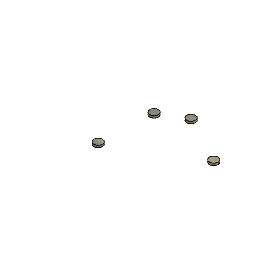
Mounting Base Magnets (Autodesk Fusion 360 design; units mm, degrees)
Autodesk Fusion 360 part; units mm, degrees
sketch "Sketch1" plane through (-0.1196, 0, 7.5625) normal (0, -1, 0) x (0.866025, 0, 0.5) in component "Magnet 1"
  circle A0 centre (26.3643, 45.4252) radius 3.7465
  arc A1 (44.7183, 43.9659) -> (15.1751, 60.8044) centre (-3.6777, -6.6091) ccw
  line L0 (15.1751, 60.8044) -> (16.1175, 64.6499)
  line L1 (16.1175, 64.6499) -> (8.0998, 66.6149)
  line L2 (8.0998, 66.6149) -> (7.1419, 62.7066)
  arc A2 (5.8468, 64.9166) -> (7.1419, 62.7066) centre (8.3868, 64.9206) ccw
  line L3 (5.8468, 64.9166) -> (5.7518, 125.1691)
  spline S0 degree 3 poles (7.7764, 127.6603) (7.4526, 127.5932) (7.1449, 127.4634) (6.5966, 127.0934) (6.3612, 126.8565) (6.0393, 126.3733) (5.9322, 126.146) (5.7879, 125.6676) (5.7514, 125.419) (5.7518, 125.1691) knots 0 0 0 0 0.099224 0.099224 0.198447 0.198447 0.273413 0.273413 0.348379 0.348379 0.348379 0.348379
  spline S1 degree 3 poles (7.7764, 127.6603) (8.1399, 127.7356) (8.4987, 127.8355) (9.8415, 128.3097) (10.758, 128.8464) (12.3456, 130.2408) (13.0009, 131.0881) (13.8928, 132.8639) (14.1662, 133.7539) (14.2925, 134.7176) (14.2982, 134.7643) (14.3035, 134.8111) knots 0.204697 0.204697 0.204697 0.204697 0.31653 0.31653 0.631913 0.631913 0.94989 0.94989 1.226398 1.226398 1.24048 1.24048 1.24048 1.24048
  spline S2 degree 3 poles (17.1425, 137.0446) (16.8143, 137.0856) (16.4812, 137.0622) (15.8428, 136.889) (15.5436, 136.7408) (15.0188, 136.3382) (14.7982, 136.0875) (14.5437, 135.6501) (14.4714, 135.4899) (14.3611, 135.157) (14.3233, 134.9853) (14.3035, 134.8111) knots 0 0 0 0 0.099224 0.099224 0.198447 0.198447 0.297671 0.297671 0.350269 0.350269 0.402867 0.402867 0.402867 0.402867
  spline S3 degree 3 poles (17.1425, 137.0446) (33.9368, 134.9438) (50.2112, 129.7725) (74.382, 116.8419) (83.022, 110.8694) (98.0523, 97.7289) (104.5331, 90.7629) (110.2478, 83.1896) knots 0.297104 0.297104 0.297104 0.297104 5.379677 5.379677 8.520913 8.520913 11.369176 11.369176 11.369176 11.369176
  spline S4 degree 3 poles (109.748, 79.6305) (110.0123, 79.8295) (110.2351, 80.0781) (110.5729, 80.6468) (110.6847, 80.9615) (110.7813, 81.6159) (110.7652, 81.9494) (110.6446, 82.4364) (110.5868, 82.5978) (110.4397, 82.9065) (110.3508, 83.0531) (110.2478, 83.1896) knots 0 0 0 0 0.099224 0.099224 0.198447 0.198447 0.297671 0.297671 0.34897 0.34897 0.400269 0.400269 0.400269 0.400269
  spline S5 degree 3 poles (109.748, 79.6305) (109.5783, 79.5028) (109.4134, 79.3683) (108.4318, 78.5028) (107.763, 77.6215) (106.8164, 75.6696) (106.5411, 74.6194) (106.4224, 72.7055) (106.4994, 71.8624) (106.7528, 70.8428) (106.8106, 70.6426) (106.8759, 70.4451) knots 0.2561 0.2561 0.2561 0.2561 0.320016 0.320016 0.648768 0.648768 0.972242 0.972242 1.225878 1.225878 1.288694 1.288694 1.288694 1.288694
  spline S6 degree 3 poles (105.7308, 67.4462) (106.0175, 67.6111) (106.2693, 67.8304) (106.6745, 68.3533) (106.8241, 68.6518) (106.979, 69.2114) (107.0097, 69.4607) (106.9974, 69.9603) (106.9544, 70.2079) (106.8759, 70.4451) knots 0 0 0 0 0.099224 0.099224 0.198447 0.198447 0.273411 0.273411 0.348375 0.348375 0.348375 0.348375
  line L4 (105.7308, 67.4462) -> (53.5032, 37.4022)
  arc A3 (50.3987, 37.8508) -> (53.5032, 37.4022) centre (52.2366, 39.6039) ccw
  line L5 (50.3987, 37.8508) -> (53.2273, 41.3906)
  line L6 (53.2273, 41.3906) -> (46.7784, 46.5439)
  line L7 (46.7784, 46.5439) -> (44.7183, 43.9659)
  circle A4 centre (114.2687, 72.6834) radius 4
  circle A5 centre (44.0521, 36.0691) radius 4
  circle A6 centre (6.0236, 135.1787) radius 4
  circle A7 centre (9.4154, 56.0666) radius 4
  arc A8 (129.4312, 70.2414) -> (-3.6777, 147.0918) centre (-3.6777, -6.6091) ccw
  line L8 (-3.6777, 147.0918) -> (-3.6777, 51.126)
  line L9 (-3.6777, 51.126) -> (46.3223, 22.2584)
  line L10 (46.3223, 22.2584) -> (129.4312, 70.2414)
  circle A9 centre (44.0521, 36.0691) radius 6.3691
  dimension "d669" = 12.7381
  constraint concentric A5 A9
  measures "d669" diameter of A9
extrude "Extrude1" add sketch "Sketch1" along normal blind 3.175 contours A5 | A9 makes body 1 in component "Magnet 1"
sketch "Sketch2" plane through (0, 0, 0) normal (0, 1, 0) x (-1, 0, 0) in component "Magnet 1"
  circle A0 centre (-19.9962, 60.8253) radius 6.3691
  circle A1 centre (-19.9962, 60.8253) radius 1.8288
  dimension "d672" = 3.6576
  constraint concentric A0 A1
  measures "d672" diameter of A1
sketch "Sketch3" plane through (0, 0, 0) normal (0, 1, 0) x (-1, 0, 0) in component "Magnet 1"
  circle A0 centre (-19.9962, 60.8253) radius 6.3691
  circle A1 centre (-44.0521, 36.0691) radius 3.683
  dimension "d675" = 7.366
  measures "d675" diameter of A1
sketch "Sketch1 (2)" plane through (-0.1196, -0.0025, 7.5625) normal (0, -1, 0) x (0.866025, 0, 0.5) in component "Magnet 1 (1)"
  circle A0 centre (26.3643, 45.4252) radius 3.7465
  arc A1 (44.7183, 43.9659) -> (15.1751, 60.8044) centre (-3.6777, -6.6091) ccw
  line L0 (15.1751, 60.8044) -> (16.1175, 64.6499)
  line L1 (16.1175, 64.6499) -> (8.0998, 66.6149)
  line L2 (8.0998, 66.6149) -> (7.1419, 62.7066)
  arc A2 (5.8468, 64.9166) -> (7.1419, 62.7066) centre (8.3868, 64.9206) ccw
  line L3 (5.8468, 64.9166) -> (5.7518, 125.1691)
  spline S0 degree 3 poles (7.7764, 127.6603) (7.4526, 127.5932) (7.1449, 127.4634) (6.5966, 127.0934) (6.3612, 126.8565) (6.0393, 126.3733) (5.9322, 126.146) (5.7879, 125.6676) (5.7514, 125.419) (5.7518, 125.1691) knots 0 0 0 0 0.099224 0.099224 0.198447 0.198447 0.273413 0.273413 0.348379 0.348379 0.348379 0.348379
  spline S1 degree 3 poles (7.7764, 127.6603) (8.1399, 127.7356) (8.4987, 127.8355) (9.8415, 128.3097) (10.758, 128.8464) (12.3456, 130.2408) (13.0009, 131.0881) (13.8928, 132.8639) (14.1662, 133.7539) (14.2925, 134.7176) (14.2982, 134.7643) (14.3035, 134.8111) knots 0.204697 0.204697 0.204697 0.204697 0.31653 0.31653 0.631913 0.631913 0.94989 0.94989 1.226398 1.226398 1.24048 1.24048 1.24048 1.24048
  spline S2 degree 3 poles (17.1425, 137.0446) (16.8143, 137.0856) (16.4812, 137.0622) (15.8428, 136.889) (15.5436, 136.7408) (15.0188, 136.3382) (14.7982, 136.0875) (14.5437, 135.6501) (14.4714, 135.4899) (14.3611, 135.157) (14.3233, 134.9853) (14.3035, 134.8111) knots 0 0 0 0 0.099224 0.099224 0.198447 0.198447 0.297671 0.297671 0.350269 0.350269 0.402867 0.402867 0.402867 0.402867
  spline S3 degree 3 poles (17.1425, 137.0446) (33.9368, 134.9438) (50.2112, 129.7725) (74.382, 116.8419) (83.022, 110.8694) (98.0523, 97.7289) (104.5331, 90.7629) (110.2478, 83.1896) knots 0.297104 0.297104 0.297104 0.297104 5.379677 5.379677 8.520913 8.520913 11.369176 11.369176 11.369176 11.369176
  spline S4 degree 3 poles (109.748, 79.6305) (110.0123, 79.8295) (110.2351, 80.0781) (110.5729, 80.6468) (110.6847, 80.9615) (110.7813, 81.6159) (110.7652, 81.9494) (110.6446, 82.4364) (110.5868, 82.5978) (110.4397, 82.9065) (110.3508, 83.0531) (110.2478, 83.1896) knots 0 0 0 0 0.099224 0.099224 0.198447 0.198447 0.297671 0.297671 0.34897 0.34897 0.400269 0.400269 0.400269 0.400269
  spline S5 degree 3 poles (109.748, 79.6305) (109.5783, 79.5028) (109.4134, 79.3683) (108.4318, 78.5028) (107.763, 77.6215) (106.8164, 75.6696) (106.5411, 74.6194) (106.4224, 72.7055) (106.4994, 71.8624) (106.7528, 70.8428) (106.8106, 70.6426) (106.8759, 70.4451) knots 0.2561 0.2561 0.2561 0.2561 0.320016 0.320016 0.648768 0.648768 0.972242 0.972242 1.225878 1.225878 1.288694 1.288694 1.288694 1.288694
  spline S6 degree 3 poles (105.7308, 67.4462) (106.0175, 67.6111) (106.2693, 67.8304) (106.6745, 68.3533) (106.8241, 68.6518) (106.979, 69.2114) (107.0097, 69.4607) (106.9974, 69.9603) (106.9544, 70.2079) (106.8759, 70.4451) knots 0 0 0 0 0.099224 0.099224 0.198447 0.198447 0.273411 0.273411 0.348375 0.348375 0.348375 0.348375
  line L4 (105.7308, 67.4462) -> (53.5032, 37.4022)
  arc A3 (50.3987, 37.8508) -> (53.5032, 37.4022) centre (52.2366, 39.6039) ccw
  line L5 (50.3987, 37.8508) -> (53.2273, 41.3906)
  line L6 (53.2273, 41.3906) -> (46.7784, 46.5439)
  line L7 (46.7784, 46.5439) -> (44.7183, 43.9659)
  circle A4 centre (114.2687, 72.6834) radius 4
  circle A5 centre (44.0521, 36.0691) radius 4
  circle A6 centre (6.0236, 135.1787) radius 4
  circle A7 centre (9.4154, 56.0666) radius 4
  arc A8 (129.4312, 70.2414) -> (-3.6777, 147.0918) centre (-3.6777, -6.6091) ccw
  line L8 (-3.6777, 147.0918) -> (-3.6777, 51.126)
  line L9 (-3.6777, 51.126) -> (46.3223, 22.2584)
  line L10 (46.3223, 22.2584) -> (129.4312, 70.2414)
  circle A9 centre (44.0521, 36.0691) radius 6.3691
  dimension "d669_1" = 12.7381
  constraint concentric A5 A9
  measures "d669_1" diameter of A9
extrude "Extrude1'" add sketch "Sketch1 (2)" along normal blind 3.175 separate body contours A5 | A9 makes body 2 in component "Magnet 1 (1)"
sketch "Sketch2 (2)" plane through (0, -0.0025, 0) normal (0, 1, 0) x (-1, 0, 0) in component "Magnet 1 (1)"
  circle A0 centre (-19.9962, 60.8253) radius 6.3691
  circle A1 centre (-19.9962, 60.8253) radius 1.8288
  dimension "d672_1" = 3.6576
  constraint concentric A0 A1
  measures "d672_1" diameter of A1
sketch "Sketch3 (2)" plane through (0, -0.0025, 0) normal (0, 1, 0) x (-1, 0, 0) in component "Magnet 1 (1)"
  circle A0 centre (-19.9962, 60.8253) radius 6.3691
  circle A1 centre (-44.0521, 36.0691) radius 3.683
  dimension "d675_1" = 7.366
  measures "d675_1" diameter of A1
sketch "Sketch1 (3)" plane through (-0.1196, -0.0025, 7.5625) normal (0, -1, 0) x (0.866025, 0, 0.5) in component "Magnet 1 (2)"
  circle A0 centre (26.3643, 45.4252) radius 3.7465
  arc A1 (44.7183, 43.9659) -> (15.1751, 60.8044) centre (-3.6777, -6.6091) ccw
  line L0 (15.1751, 60.8044) -> (16.1175, 64.6499)
  line L1 (16.1175, 64.6499) -> (8.0998, 66.6149)
  line L2 (8.0998, 66.6149) -> (7.1419, 62.7066)
  arc A2 (5.8468, 64.9166) -> (7.1419, 62.7066) centre (8.3868, 64.9206) ccw
  line L3 (5.8468, 64.9166) -> (5.7518, 125.1691)
  spline S0 degree 3 poles (7.7764, 127.6603) (7.4526, 127.5932) (7.1449, 127.4634) (6.5966, 127.0934) (6.3612, 126.8565) (6.0393, 126.3733) (5.9322, 126.146) (5.7879, 125.6676) (5.7514, 125.419) (5.7518, 125.1691) knots 0 0 0 0 0.099224 0.099224 0.198447 0.198447 0.273413 0.273413 0.348379 0.348379 0.348379 0.348379
  spline S1 degree 3 poles (7.7764, 127.6603) (8.1399, 127.7356) (8.4987, 127.8355) (9.8415, 128.3097) (10.758, 128.8464) (12.3456, 130.2408) (13.0009, 131.0881) (13.8928, 132.8639) (14.1662, 133.7539) (14.2925, 134.7176) (14.2982, 134.7643) (14.3035, 134.8111) knots 0.204697 0.204697 0.204697 0.204697 0.31653 0.31653 0.631913 0.631913 0.94989 0.94989 1.226398 1.226398 1.24048 1.24048 1.24048 1.24048
  spline S2 degree 3 poles (17.1425, 137.0446) (16.8143, 137.0856) (16.4812, 137.0622) (15.8428, 136.889) (15.5436, 136.7408) (15.0188, 136.3382) (14.7982, 136.0875) (14.5437, 135.6501) (14.4714, 135.4899) (14.3611, 135.157) (14.3233, 134.9853) (14.3035, 134.8111) knots 0 0 0 0 0.099224 0.099224 0.198447 0.198447 0.297671 0.297671 0.350269 0.350269 0.402867 0.402867 0.402867 0.402867
  spline S3 degree 3 poles (17.1425, 137.0446) (33.9368, 134.9438) (50.2112, 129.7725) (74.382, 116.8419) (83.022, 110.8694) (98.0523, 97.7289) (104.5331, 90.7629) (110.2478, 83.1896) knots 0.297104 0.297104 0.297104 0.297104 5.379677 5.379677 8.520913 8.520913 11.369176 11.369176 11.369176 11.369176
  spline S4 degree 3 poles (109.748, 79.6305) (110.0123, 79.8295) (110.2351, 80.0781) (110.5729, 80.6468) (110.6847, 80.9615) (110.7813, 81.6159) (110.7652, 81.9494) (110.6446, 82.4364) (110.5868, 82.5978) (110.4397, 82.9065) (110.3508, 83.0531) (110.2478, 83.1896) knots 0 0 0 0 0.099224 0.099224 0.198447 0.198447 0.297671 0.297671 0.34897 0.34897 0.400269 0.400269 0.400269 0.400269
  spline S5 degree 3 poles (109.748, 79.6305) (109.5783, 79.5028) (109.4134, 79.3683) (108.4318, 78.5028) (107.763, 77.6215) (106.8164, 75.6696) (106.5411, 74.6194) (106.4224, 72.7055) (106.4994, 71.8624) (106.7528, 70.8428) (106.8106, 70.6426) (106.8759, 70.4451) knots 0.2561 0.2561 0.2561 0.2561 0.320016 0.320016 0.648768 0.648768 0.972242 0.972242 1.225878 1.225878 1.288694 1.288694 1.288694 1.288694
  spline S6 degree 3 poles (105.7308, 67.4462) (106.0175, 67.6111) (106.2693, 67.8304) (106.6745, 68.3533) (106.8241, 68.6518) (106.979, 69.2114) (107.0097, 69.4607) (106.9974, 69.9603) (106.9544, 70.2079) (106.8759, 70.4451) knots 0 0 0 0 0.099224 0.099224 0.198447 0.198447 0.273411 0.273411 0.348375 0.348375 0.348375 0.348375
  line L4 (105.7308, 67.4462) -> (53.5032, 37.4022)
  arc A3 (50.3987, 37.8508) -> (53.5032, 37.4022) centre (52.2366, 39.6039) ccw
  line L5 (50.3987, 37.8508) -> (53.2273, 41.3906)
  line L6 (53.2273, 41.3906) -> (46.7784, 46.5439)
  line L7 (46.7784, 46.5439) -> (44.7183, 43.9659)
  circle A4 centre (114.2687, 72.6834) radius 4
  circle A5 centre (44.0521, 36.0691) radius 4
  circle A6 centre (6.0236, 135.1787) radius 4
  circle A7 centre (9.4154, 56.0666) radius 4
  arc A8 (129.4312, 70.2414) -> (-3.6777, 147.0918) centre (-3.6777, -6.6091) ccw
  line L8 (-3.6777, 147.0918) -> (-3.6777, 51.126)
  line L9 (-3.6777, 51.126) -> (46.3223, 22.2584)
  line L10 (46.3223, 22.2584) -> (129.4312, 70.2414)
  circle A9 centre (44.0521, 36.0691) radius 6.3691
  dimension "d669_2" = 12.7381
  constraint concentric A5 A9
  measures "d669_2" diameter of A9
extrude "Extrude1''" add sketch "Sketch1 (3)" along normal blind 3.175 separate body contours A5 | A9 makes body 3 in component "Magnet 1 (2)"
sketch "Sketch2 (3)" plane through (0, -0.0025, 0) normal (0, 1, 0) x (-1, 0, 0) in component "Magnet 1 (2)"
  circle A0 centre (-19.9962, 60.8253) radius 6.3691
  circle A1 centre (-19.9962, 60.8253) radius 1.8288
  dimension "d672_2" = 3.6576
  constraint concentric A0 A1
  measures "d672_2" diameter of A1
sketch "Sketch3 (3)" plane through (0, -0.0025, 0) normal (0, 1, 0) x (-1, 0, 0) in component "Magnet 1 (2)"
  circle A0 centre (-19.9962, 60.8253) radius 6.3691
  circle A1 centre (-44.0521, 36.0691) radius 3.683
  dimension "d675_2" = 7.366
  measures "d675_2" diameter of A1
sketch "Sketch1 (4)" plane through (-0.1196, -0.0025, 7.5625) normal (0, -1, 0) x (0.866025, 0, 0.5) in component "Magnet 1 (3)"
  circle A0 centre (26.3643, 45.4252) radius 3.7465
  arc A1 (44.7183, 43.9659) -> (15.1751, 60.8044) centre (-3.6777, -6.6091) ccw
  line L0 (15.1751, 60.8044) -> (16.1175, 64.6499)
  line L1 (16.1175, 64.6499) -> (8.0998, 66.6149)
  line L2 (8.0998, 66.6149) -> (7.1419, 62.7066)
  arc A2 (5.8468, 64.9166) -> (7.1419, 62.7066) centre (8.3868, 64.9206) ccw
  line L3 (5.8468, 64.9166) -> (5.7518, 125.1691)
  spline S0 degree 3 poles (7.7764, 127.6603) (7.4526, 127.5932) (7.1449, 127.4634) (6.5966, 127.0934) (6.3612, 126.8565) (6.0393, 126.3733) (5.9322, 126.146) (5.7879, 125.6676) (5.7514, 125.419) (5.7518, 125.1691) knots 0 0 0 0 0.099224 0.099224 0.198447 0.198447 0.273413 0.273413 0.348379 0.348379 0.348379 0.348379
  spline S1 degree 3 poles (7.7764, 127.6603) (8.1399, 127.7356) (8.4987, 127.8355) (9.8415, 128.3097) (10.758, 128.8464) (12.3456, 130.2408) (13.0009, 131.0881) (13.8928, 132.8639) (14.1662, 133.7539) (14.2925, 134.7176) (14.2982, 134.7643) (14.3035, 134.8111) knots 0.204697 0.204697 0.204697 0.204697 0.31653 0.31653 0.631913 0.631913 0.94989 0.94989 1.226398 1.226398 1.24048 1.24048 1.24048 1.24048
  spline S2 degree 3 poles (17.1425, 137.0446) (16.8143, 137.0856) (16.4812, 137.0622) (15.8428, 136.889) (15.5436, 136.7408) (15.0188, 136.3382) (14.7982, 136.0875) (14.5437, 135.6501) (14.4714, 135.4899) (14.3611, 135.157) (14.3233, 134.9853) (14.3035, 134.8111) knots 0 0 0 0 0.099224 0.099224 0.198447 0.198447 0.297671 0.297671 0.350269 0.350269 0.402867 0.402867 0.402867 0.402867
  spline S3 degree 3 poles (17.1425, 137.0446) (33.9368, 134.9438) (50.2112, 129.7725) (74.382, 116.8419) (83.022, 110.8694) (98.0523, 97.7289) (104.5331, 90.7629) (110.2478, 83.1896) knots 0.297104 0.297104 0.297104 0.297104 5.379677 5.379677 8.520913 8.520913 11.369176 11.369176 11.369176 11.369176
  spline S4 degree 3 poles (109.748, 79.6305) (110.0123, 79.8295) (110.2351, 80.0781) (110.5729, 80.6468) (110.6847, 80.9615) (110.7813, 81.6159) (110.7652, 81.9494) (110.6446, 82.4364) (110.5868, 82.5978) (110.4397, 82.9065) (110.3508, 83.0531) (110.2478, 83.1896) knots 0 0 0 0 0.099224 0.099224 0.198447 0.198447 0.297671 0.297671 0.34897 0.34897 0.400269 0.400269 0.400269 0.400269
  spline S5 degree 3 poles (109.748, 79.6305) (109.5783, 79.5028) (109.4134, 79.3683) (108.4318, 78.5028) (107.763, 77.6215) (106.8164, 75.6696) (106.5411, 74.6194) (106.4224, 72.7055) (106.4994, 71.8624) (106.7528, 70.8428) (106.8106, 70.6426) (106.8759, 70.4451) knots 0.2561 0.2561 0.2561 0.2561 0.320016 0.320016 0.648768 0.648768 0.972242 0.972242 1.225878 1.225878 1.288694 1.288694 1.288694 1.288694
  spline S6 degree 3 poles (105.7308, 67.4462) (106.0175, 67.6111) (106.2693, 67.8304) (106.6745, 68.3533) (106.8241, 68.6518) (106.979, 69.2114) (107.0097, 69.4607) (106.9974, 69.9603) (106.9544, 70.2079) (106.8759, 70.4451) knots 0 0 0 0 0.099224 0.099224 0.198447 0.198447 0.273411 0.273411 0.348375 0.348375 0.348375 0.348375
  line L4 (105.7308, 67.4462) -> (53.5032, 37.4022)
  arc A3 (50.3987, 37.8508) -> (53.5032, 37.4022) centre (52.2366, 39.6039) ccw
  line L5 (50.3987, 37.8508) -> (53.2273, 41.3906)
  line L6 (53.2273, 41.3906) -> (46.7784, 46.5439)
  line L7 (46.7784, 46.5439) -> (44.7183, 43.9659)
  circle A4 centre (114.2687, 72.6834) radius 4
  circle A5 centre (44.0521, 36.0691) radius 4
  circle A6 centre (6.0236, 135.1787) radius 4
  circle A7 centre (9.4154, 56.0666) radius 4
  arc A8 (129.4312, 70.2414) -> (-3.6777, 147.0918) centre (-3.6777, -6.6091) ccw
  line L8 (-3.6777, 147.0918) -> (-3.6777, 51.126)
  line L9 (-3.6777, 51.126) -> (46.3223, 22.2584)
  line L10 (46.3223, 22.2584) -> (129.4312, 70.2414)
  circle A9 centre (44.0521, 36.0691) radius 6.3691
  dimension "d669_3" = 12.7381
  constraint concentric A5 A9
  measures "d669_3" diameter of A9
extrude "Extrude1'''" add sketch "Sketch1 (4)" along normal blind 3.175 separate body contours A5 | A9 makes body 4 in component "Magnet 1 (3)"
sketch "Sketch2 (4)" plane through (0, -0.0025, 0) normal (0, 1, 0) x (-1, 0, 0) in component "Magnet 1 (3)"
  circle A0 centre (-19.9962, 60.8253) radius 6.3691
  circle A1 centre (-19.9962, 60.8253) radius 1.8288
  dimension "d672_3" = 3.6576
  constraint concentric A0 A1
  measures "d672_3" diameter of A1
sketch "Sketch3 (4)" plane through (0, -0.0025, 0) normal (0, 1, 0) x (-1, 0, 0) in component "Magnet 1 (3)"
  circle A0 centre (-19.9962, 60.8253) radius 6.3691
  circle A1 centre (-44.0521, 36.0691) radius 3.683
  dimension "d675_3" = 7.366
  measures "d675_3" diameter of A1
component "Magnet 1" placed x (1, 0, 0) y (0, 1, 0) z (0, 0, 1) at (0, 0, 0)
component "Magnet 1 (1)" placed x (1, 0, 0) y (0, 1, 0) z (0, 0, 1) at (-34.6367, 0, 19.9975)
component "Magnet 1 (2)" placed x (1, 0, 0) y (0, 1, 0) z (0, 0, 1) at (70.2165, 0, 36.6143)
component "Magnet 1 (3)" placed x (1, 0, 0) y (0, 1, 0) z (0, 0, 1) at (-38.0285, 0, 99.1096)
